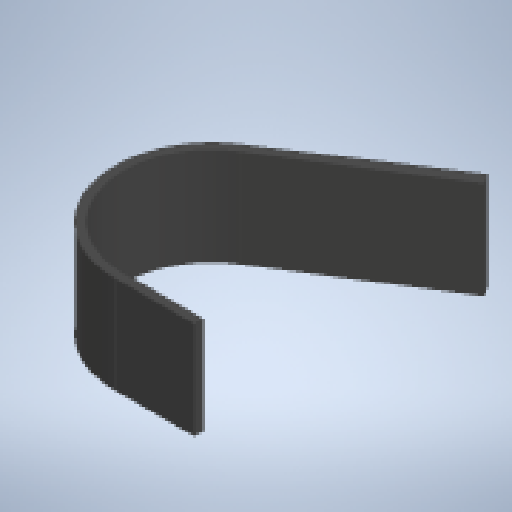
# Autodesk Inventor part: bend_sensor
Saved by Autodesk Inventor 2025.2 (Build 292293000, 293)
## iProperties
Created: 2025-06-25
Part Number: bend_sensor
Material: 一般
Document SubType Name: Modeling
Designer: naka6
Density: 1 g/cm^3
Appearance: 既定
Author: naka6
Autodesk Inventor part; units mm, degrees
ref_plane "YZ Plane" through (0, 0, 0) normal (1, 0, 0) x (0, 1, 0)
ref_plane "XZ Plane" through (0, 0, 0) normal (0, 1, 0) x (-1, 0, 0)
ref_plane "XY Plane" through (0, 0, 0) normal (0, 0, 1) x (1, 0, 0)
sketch "スケッチ1" plane through (0, 0, 0) normal (0, 1, 0) x (-1, 0, 0)
  line L0 (0, 0) -> (-15, 0)
  line L1 (-15, 0) -> (-15, 0.5)
  line L2 (-15, 0.5) -> (0, 0.5)
  line L3 (0, 0.5) -> (0, 0)
  circle A0 centre (0, -5) radius 5
  circle A1 centre (0, -5) radius 5.5
  line L4 (1.2941, -9.8296) -> (-32.5133, -18.8883)
  line L5 (-32.5133, -18.8883) -> (-32.3839, -19.3713)
  line L6 (-32.3839, -19.3713) -> (1.4235, -10.3126)
  point P0 (-0.2935, -9.9914)
  point P1 (-0.9191, -10.4227)
  point P2 (-2.2913, 0)
  dimension "d3" = 10
  dimension "d2" = 11
  dimension "d4" = 15
  dimension "d5" = 35
  dimension "d6" = 15
  constraints: 14 end point, 3 perpendicular, 2 horizontal, 2 parallel, 2 point on circle, 2 tangent, 1 centre point, 1 coincident, 4 other
  measures "d2" diameter of A1
  measures "d4" distance of L1.end L2.end
  measures "d5" distance of L5.end L6.end
  measures "d6" angle of L1 L5
extrude "押し出し1" add sketch "スケッチ1" along normal blind 5 contours L0 A1 L3 | L3 A1 L4 A0 | L0 L1 L2 A1 | A1 L6 L5 L4
